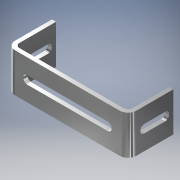
# Autodesk Inventor part: thumbkey_cup
Saved by Autodesk Inventor 2018 (Build 220112000, 112)
## iProperties
Created: 2018-04-06
Part Number: thumbkey_cup
Material: アルミニウム 6061
Document SubType Name: Sheet Metal
Designer: NaMACHAN
Density: 2.7 g/cm^3
Sheet Metal Rule: Default_mm
Appearance: アルミニウム - フラット
Mass: 27.9111 g
Surface Area: 87.5065 cm^2
Volume: 10.3374 cm^3
Flat Pattern Width: 1.9 cm
Flat Pattern Length: 9.60478 cm
Flat Pattern Area: 18.2491 cm^2
Sheet Metal Width: 19.000 mm
Sheet Metal Length: 96.048 mm
Sheet Metal Area: 1824.908 mm^2
Author: NaMACHAN
Autodesk Inventor part; units mm, degrees
ref_plane "YZ Plane" through (0, 0, 0) normal (1, 0, 0) x (0, 1, 0)
ref_plane "XZ Plane" through (0, 0, 0) normal (0, 1, 0) x (-1, 0, 0)
ref_plane "XY Plane" through (0, 0, 0) normal (0, 0, 1) x (1, 0, 0)
sketch "スケッチ1" plane through (0, 0, 0) normal (0, 1, 0) x (-1, 0, 0)
  line L0 (-27.5, -9.5) -> (27.5, -9.5)
  line L1 (27.5, -9.5) -> (27.5, 9.5)
  line L2 (27.5, 9.5) -> (-27.5, 9.5)
  line L3 (-27.5, 9.5) -> (-27.5, -9.5)
  line L4 (-27.5, -9.5) -> (27.5, 9.5) construction
  line L5 (27.5, -9.5) -> (-27.5, 9.5) construction
  point P0 (0, 0)
  dimension "d0" = 19
  dimension "d1" = 55
  measures "d0" distance of L0.end L1.end
  measures "d1" distance of L0.start L0.end
extrude "プレート1" add sketch "スケッチ1" along normal blind 2
sketch "スケッチ2" plane through (27.5, 0, 9.5) normal (1, 0, 0) x (0, 0, -1)
  line L0 (0, 2) -> (19, 2)
  line L1 (19, 2) -> (0, 2)
  line L2 (0, 2) -> (0, 22)
  line L3 (0, 22) -> (19, 22)
  line L4 (19, 22) -> (19, 2)
  point P0 (9.5, 0)
  dimension "d3" = 20
  measures "d3" distance of L3.end L0.end
sheet face with bend "面2" sketch "スケッチ2" thickness 2 toward (1, 0, 0) bend radius 2
bend "曲げ1"
sketch "スケッチ3" plane through (-27.5, 0, -9.5) normal (-1, 0, 0) x (0, 0, 1)
  line L0 (0, 0) -> (0, 2)
  line L1 (0, 22) -> (19, 22)
  line L2 (0, 2) -> (19, 2)
  line L3 (19, 2) -> (19, 22)
  line L4 (19, 22) -> (0, 22)
  line L5 (0, 22) -> (0, 2)
  point P0 (9.5, 0)
sheet face with bend "面3" sketch "スケッチ3" thickness 2 toward (-1, 0, 0) bend radius 2
bend "曲げ2"
sketch "スケッチ4" plane through (-29.5, 0, -9.5) normal (-1, 0, 0) x (0, 0, 1)
  line L0 (7.5, 18) -> (7.5, 8)
  arc A0 (7.5, 8) -> (11.5, 8) centre (9.5, 8) ccw
  line L1 (11.5, 8) -> (11.5, 18)
  arc A1 (11.5, 18) -> (7.5, 18) centre (9.5, 18) ccw
  line L2 (19, 22) -> (19, 4) projected
  line L3 (0, 22) -> (19, 22) projected
  line L4 (19, 4) -> (0, 4) projected
  point P0 (9.5, 0)
  dimension "d18" = 2
  dimension "d33" = 4
  dimension "d34" = 4
  constraints: 4 end point, 4 point on circle, 4 tangent, 2 centre point, 1 parallel, 1 vertical, 1 vertical alignment
  measures "d18" radius of A1
  measures "d33" distance from line of L3 A1.centre
  measures "d34" distance from line of L4 A0.centre
extrude "押し出し1" cut sketch "スケッチ4" against normal blind 100
sketch "スケッチ5" plane through (0, 2, 0) normal (0, 1, 0) x (1, 0, 0)
  line L0 (-19.5, -2) -> (19.5, -2)
  arc A0 (19.5, -2) -> (19.5, 2) centre (19.5, 0) ccw
  line L1 (19.5, 2) -> (-19.5, 2)
  arc A1 (-19.5, 2) -> (-19.5, -2) centre (-19.5, 0) ccw
  line L2 (25.5, -9.5) -> (-25.5, -9.5) projected
  line L3 (-25.5, 9.5) -> (-25.5, -9.5) projected
  line L4 (25.5, -9.5) -> (25.5, 9.5) projected
  point P0 (0, 0)
  point P1 (-21.5, 0)
  dimension "d22" = 2
  dimension "d35" = 6
  dimension "d36" = 6
  constraints: 5 point on circle, 4 end point, 4 tangent, 2 centre point, 1 horizontal, 1 horizontal alignment, 1 parallel
  measures "d22" radius of A1
  measures "d35" distance from line of L3 A1.centre
  measures "d36" distance from line of L4 A0.centre
extrude "押し出し2" cut sketch "スケッチ5" against normal blind 3
equation "\"d2\" = Thickness"
equation "\"d4\" = BendRadius"
equation "\"d5\" = BendReliefWidth"
equation "\"d7\" = MinimumRemnant"
equation "\"d6\" = BendReliefDepth"
equation "\"d8\" = TransitionRadius"
equation "\"d9\" = BendRadius"
equation "\"d10\" = BendReliefWidth"
equation "\"d12\" = MinimumRemnant"
equation "\"d11\" = BendReliefDepth"
equation "\"d13\" = TransitionRadius"
equation "\"BendRadius\" = Thickness"
equation "\"BendReliefWidth\" = Thickness"
equation "\"BendReliefDepth\" = 0.5 * Thickness"
equation "\"CornerReliefSize\" = 4 * Thickness"
equation "\"MinimumRemnant\" = 2 * Thickness"
equation "\"TransitionRadius\" = BendRadius"
equation "\"JacobiRadiusSize\" = BendRadius"
equation "\"GapSize\" = Thickness"
equation "\"Thickness\" = 2"
